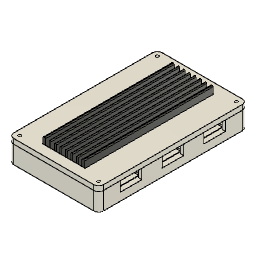
TLSmootherBox_v17 (Autodesk Fusion 360 design; units mm, degrees)
Autodesk Fusion 360 part; units mm, degrees
sketch "Sketch1" plane through (0, 0, 0) normal (0, 0, 1) x (1, 0, 0) in component "Base"
  line L0 (0, 108.9935) -> (0, -108.9935) construction
  line L1 (-168.2514, 0) -> (168.2514, 0) construction
  line L2 (37.875, 24.125) -> (-37.875, 24.125)
  line L3 (-37.875, 24.125) -> (-37.875, -24.125)
  line L4 (-37.875, -24.125) -> (37.875, -24.125)
  line L5 (37.875, -24.125) -> (37.875, 24.125)
  line L6 (37.875, 24.125) -> (-37.875, -24.125) construction
  line L7 (-37.875, 24.125) -> (37.875, -24.125) construction
  line L8 (-42.875, 25.125) -> (42.875, 25.125)
  line L9 (42.875, 25.125) -> (42.875, -25.125)
  line L10 (42.875, -25.125) -> (-42.875, -25.125)
  line L11 (-42.875, -25.125) -> (-42.875, 25.125)
  line L12 (44.875, -27.125) -> (-44.875, -27.125)
  line L13 (-44.875, -27.125) -> (-44.875, 27.125)
  line L14 (-44.875, 27.125) -> (44.875, 27.125)
  line L15 (44.875, 27.125) -> (44.875, -27.125)
  circle A0 centre (-41.625, 23.875) radius 0.875
  circle A1 centre (41.625, 23.875) radius 0.875
  circle A2 centre (-41.625, -23.875) radius 0.875
  circle A3 centre (41.625, -23.875) radius 0.875
  line L16 (-44.875, 27.125) -> (-38.875, 27.125)
  line L17 (-38.875, 27.125) -> (-38.875, 21.125)
  line L18 (-38.875, 21.125) -> (-44.875, 21.125)
  line L19 (-44.875, 21.125) -> (-44.875, 27.125)
  line L20 (38.875, 21.125) -> (44.875, 21.125)
  line L21 (38.875, 27.125) -> (38.875, 21.125)
  line L22 (-38.875, -21.125) -> (-44.875, -21.125)
  line L23 (-38.875, -27.125) -> (-38.875, -21.125)
  line L24 (38.875, -27.125) -> (38.875, -21.125)
  line L25 (38.875, -21.125) -> (44.875, -21.125)
  line L26 (-37.875, 22.125) -> (37.875, 22.125)
  line L27 (-37.875, -22.125) -> (37.875, -22.125)
  line L28 (-35.875, 24.125) -> (-35.875, -24.125)
  line L29 (-12.625, 24.125) -> (-12.625, -24.125)
  line L30 (-14.625, 24.125) -> (-14.625, -24.125)
  circle A4 centre (-41.625, 23.875) radius 1.25
  circle A5 centre (41.625, 23.875) radius 1.25
  circle A6 centre (-41.625, -23.875) radius 1.25
  circle A7 centre (41.625, -23.875) radius 1.25
  dimension "d9" = 48.25
  dimension "d11" = 75.75
  dimension "d14" = 1
  dimension "d15" = 5
  dimension "d36" = 1.75
  dimension "d83" = 0
  dimension "d84" = 0
  dimension "d85" = 0
  dimension "d86" = 0
  dimension "d95" = 0
  dimension "d96" = 0
  dimension "d97" = 0
  dimension "d98" = 0
  dimension "d103" = 0
  dimension "d104" = 0
  dimension "d105" = 0
  dimension "d106" = 0
  dimension "d134" = 0
  dimension "d135" = 0
  dimension "d136" = 0
  dimension "d137" = 0
  dimension "d147" = 21.125
  dimension "d148" = 38.875
  dimension "d149" = 41.625
  dimension "d150" = 23.875
  dimension "d154" = 2
  dimension "d160" = 2
  dimension "d161" = 25.25
  dimension "d162" = 2
  dimension "d188" = 0
  dimension "d189" = 0
  dimension "d190" = 0
  dimension "d191" = 0
  dimension "d240" = 2.5
  constraint horizontal L1
  constraint perpendicular L2 L3
  constraint parallel L2 L4
  constraint parallel L3 L5
  constraint horizontal L2
  constraint coincident L6 origin
  constraint coincident L7 origin
  constraint horizontal L8
  constraint vertical L9
  constraint horizontal L10
  constraint vertical L11
  constraint symmetric L1 L8 L10
  constraint symmetric L0 L9 L11
  constraint midpoint L0 origin
  constraint midpoint origin L1
  constraint symmetric L0 A0 A1
  constraint symmetric L1 A0 A2
  constraint symmetric L1 A1 A3
  constraint horizontal L16
  constraint vertical L17
  constraint horizontal L18
  constraint vertical L19
  constraint symmetric L0 L16.end L21.start
  constraint symmetric L0 L17.end L20.start
  constraint symmetric L0 L18.end L20.end
  constraint symmetric L1 L16.end L23.start
  constraint symmetric L1 L17.end L22.start
  constraint symmetric L1 L18.end L22.end
  constraint symmetric L1 L20.start L24.end
  constraint symmetric L1 L20.end L25.end
  constraint symmetric L1 L21.start L24.start
  constraint coincident L3 L26.start
  constraint coincident L5 L26.end
  constraint perpendicular L5 L26
  constraint coincident L3 L27.start
  constraint coincident L5 L27.end
  constraint perpendicular L5 L27
  constraint symmetric L1 L26 L27
  constraint coincident L2 L28.start
  constraint coincident L4 L28.end
  constraint perpendicular L4 L28
  constraint coincident L2 L29.start
  constraint coincident L4 L29.end
  constraint perpendicular L4 L29
  constraint coincident L2 L30.start
  constraint coincident L4 L30.end
  constraint perpendicular L4 L30
  constraint concentric A0 A4
  constraint symmetric L0 A4 A5
  constraint symmetric L1 A4 A6
  constraint symmetric L1 A5 A7
  measures "d9" distance of L2 L4
  measures "d11" distance of L3 L5
  measures "d14" distance of L2 L8
  measures "d15" distance of L3 L11
  measures "d36" diameter of A0
  measures "d147" distance of L1 L18
  measures "d148" distance of L0 L17
  measures "d149" distance of L0 A0.centre
  measures "d150" distance of L1 A0.centre
  measures "d154" distance of L2 L26
  measures "d160" distance of L3 L28
  measures "d161" distance of L3 L29
  measures "d162" distance of L29 L30
  measures "d240" diameter of A4
extrude "Extrude1" add sketch "Sketch1" along normal blind 2 contours L2 L5 L26 L29 | L2 L26 L29 L30 | L5 L26 L27 L29 | L2 L26 L28 L30 | L26 L27 L29 L30 | L4 L5 L27 L29 | L2 L3 L26 L28 | L26 L27 L28 L30 | L4 L27 L29 L30 | L3 L26 L27 L28 | L4 L27 L28 L30 | L3 L4 L27 L28 | L8 L11 L13 L14 L16 L17 L18 L19 | L8 L11 A4 | L8 L11 L17 L18 A4 | A4 | L8 L14 L17 L21 | L8 L9 L10 L11 L17 L18 L20 L21 L22 L23 L24 L25 | L11 L13 L18 L22 | L8 L9 L14 L15 L20 L21 | L8 L9 L20 L21 A5 | L10 L11 L22 L23 A6 | L10 L11 L12 L13 L22 L23 | L8 L9 A5 | A5 | L10 L11 A6 | A6 | L9 L15 L20 L25 | L10 L12 L23 L24 | L9 L10 L12 L15 L24 L25 | L9 L10 L24 L25 A7 | A7 | L9 L10 A7 | A0 | A1 | A2 | A3 makes body 1 in component "Base"
extrude "Extrude2" add sketch "Sketch1" along normal blind 10.75 contours L8 L11 L13 L14 L16 L17 L18 L19 | L8 L11 A4 | L8 L11 L17 L18 A4 | A4 | L8 L14 L17 L21 | L11 L13 L18 L22 | L8 L9 L14 L15 L20 L21 | L8 L9 L20 L21 A5 | L10 L11 L22 L23 A6 | L10 L11 L12 L13 L22 L23 | L8 L9 A5 | A5 | L10 L11 A6 | A6 | L9 L15 L20 L25 | L10 L12 L23 L24 | L9 L10 L12 L15 L24 L25 | L9 L10 L24 L25 A7 | A7 | L9 L10 A7 | A0 | A1 | A2 | A3 bodies 1 in component "Base"
extrude "Extrude5" cut sketch "Sketch1" against normal blind 6 from surface at 10.75 contours A4 | A5 | A6 | A7 | A0 | A1 | A2 | A3 bodies 1 in component "Base"
extrude "Extrude4" add sketch "Sketch1" along normal blind 2.75 from surface at 2 contours L8 L11 A4 | L8 L11 L17 L18 A4 | A4 | L8 L9 L10 L11 L17 L18 L20 L21 L22 L23 L24 L25 | L8 L9 L20 L21 A5 | L10 L11 L22 L23 A6 | L8 L9 A5 | A5 | L10 L11 A6 | A6 | L9 L10 L24 L25 A7 | A7 | L9 L10 A7 | A0 | A1 | A2 | A3 bodies 1 in component "Base"
extrude "Extrude3" add sketch "Sketch1" along normal blind 1 from surface at 2 contours L2 L26 L29 L30 | L2 L26 L28 L30 | L26 L27 L29 L30 | L2 L3 L26 L28 | L4 L27 L29 L30 | L3 L26 L27 L28 | L4 L27 L28 L30 | L3 L4 L27 L28 bodies 1 in component "Base"
pattern_linear "R-Pattern2" count 3 spacing 25.25 along (1, 0, 0) of "Extrude3" in component "Base"
fillet "Fillet1" radius 3 4 edges at (44.875, -27.125, 5.375) (-44.875, -27.125, 5.375) (-44.875, 27.125, 5.375) (44.875, 27.125, 5.375) on bodies 1 in component "Base"
fillet "Fillet2" radius 2 4 edges at (-38.875, 21.125, 7.75) (38.875, 21.125, 7.75) (-38.875, -21.125, 7.75) (38.875, -21.125, 7.75) on bodies 1 in component "Base"
fillet "Fillet3" radius 0.5 8 edges at (-42.875, -21.125, 7.75) (-38.875, -25.125, 7.75) (38.875, -25.125, 7.75) (42.875, -21.125, 7.75) (38.875, 25.125, 7.75) (42.875, 21.125, 7.75) (-42.875, 21.125, 7.75) (-38.875, 25.125, 7.75) on bodies 1 in component "Base"
sketch "Sketch2" plane through (0, -27.125, 0) normal (0, -1, 0) x (1, 0, 0) in component "Base"
  line L0 (-41.875, 10.75) -> (-41.875, 0)
  line L1 (-41.875, 0) -> (41.875, 0)
  line L2 (41.875, 0) -> (41.875, 10.75)
  line L3 (41.875, 10.75) -> (-41.875, 10.75)
  line L4 (0, 68.7375) -> (0, -68.7375) construction
  line L5 (37.875, 3) -> (-37.875, 3)
  line L6 (-37.875, 3) -> (-37.875, 4.75)
  line L7 (-37.875, 4.75) -> (37.875, 4.75)
  line L8 (37.875, 4.75) -> (37.875, 3)
  line L9 (-31.75, 10.75) -> (-31.75, 4.75)
  line L10 (-18.75, 10.75) -> (-18.75, 4.75)
  dimension "d167" = 6.125
  dimension "d168" = 13
  constraint vertical L4
  constraint midpoint L4 origin
  constraint coincident L3 L9.start
  constraint coincident L7 L9.end
  constraint perpendicular L7 L9
  constraint coincident L3 L10.start
  constraint coincident L7 L10.end
  constraint perpendicular L7 L10
  measures "d167" distance of L6 L9
  measures "d168" distance of L9 L10
extrude "Extrude6" cut sketch "Sketch2" against normal through all contours L3 L7 L9 L10 bodies 1 in component "Base"
pattern_linear "R-Pattern1" count 3 spacing 25.25 along (1, 0, 0) of "Extrude6" in component "Base"
sketch "Sketch1 (2)" plane through (0, 0, 2) normal (0, 0, 1) x (1, 0, 0) in component "Lid"
  line L0 (-31.75, 27.125) -> (-41.875, 27.125)
  arc A0 (-41.875, 27.125) -> (-44.875, 24.125) centre (-41.875, 24.125) ccw
  line L1 (-44.875, 24.125) -> (-44.875, -24.125)
  arc A1 (-44.875, -24.125) -> (-41.875, -27.125) centre (-41.875, -24.125) ccw
  line L2 (-41.875, -27.125) -> (-31.75, -27.125)
  line L3 (-31.75, -25.125) -> (-38.375, -25.125)
  line L4 (-42.875, -20.625) -> (-42.875, 20.625)
  line L5 (-38.375, 25.125) -> (-31.75, 25.125)
  line L6 (31.75, -27.125) -> (41.875, -27.125)
  arc A2 (41.875, -27.125) -> (44.875, -24.125) centre (41.875, -24.125) ccw
  line L7 (44.875, -24.125) -> (44.875, 24.125)
  arc A3 (44.875, 24.125) -> (41.875, 27.125) centre (41.875, 24.125) ccw
  line L8 (41.875, 27.125) -> (31.75, 27.125)
  line L9 (31.75, 25.125) -> (38.375, 25.125)
  line L10 (42.875, 20.625) -> (42.875, -20.625)
  line L11 (38.375, -25.125) -> (31.75, -25.125)
  line L12 (31.75, -25.125) -> (38.375, -25.125)
  line L13 (42.875, -20.625) -> (42.875, 20.625)
  line L14 (-42.875, 20.625) -> (-42.875, -20.625)
  line L15 (0, 108.9935) -> (0, -108.9935) construction
  line L16 (-168.2514, 0) -> (168.2514, 0) construction
  line L17 (37.875, -24.125) -> (37.875, 24.125)
  line L18 (37.875, 24.125) -> (-37.875, 24.125)
  line L19 (-37.875, 24.125) -> (-37.875, -24.125)
  line L20 (-37.875, -24.125) -> (37.875, -24.125)
  arc A4 (-38.875, -24.625) -> (-38.375, -25.125) centre (-38.375, -24.625) ccw
  line L21 (-38.875, -24.625) -> (-38.875, -23.125)
  arc A5 (-38.875, -23.125) -> (-40.875, -21.125) centre (-40.875, -23.125) ccw
  line L22 (-40.875, -21.125) -> (-42.375, -21.125)
  arc A6 (-42.875, -20.625) -> (-42.375, -21.125) centre (-42.375, -20.625) ccw
  arc A7 (-42.375, 21.125) -> (-42.875, 20.625) centre (-42.375, 20.625) ccw
  line L23 (-42.375, 21.125) -> (-40.875, 21.125)
  arc A8 (-40.875, 21.125) -> (-38.875, 23.125) centre (-40.875, 23.125) ccw
  line L24 (-38.875, 23.125) -> (-38.875, 24.625)
  arc A9 (-38.375, 25.125) -> (-38.875, 24.625) centre (-38.375, 24.625) ccw
  arc A10 (38.875, 24.625) -> (38.375, 25.125) centre (38.375, 24.625) ccw
  line L25 (38.875, 24.625) -> (38.875, 23.125)
  arc A11 (38.875, 23.125) -> (40.875, 21.125) centre (40.875, 23.125) ccw
  line L26 (40.875, 21.125) -> (42.375, 21.125)
  arc A12 (42.875, 20.625) -> (42.375, 21.125) centre (42.375, 20.625) ccw
  arc A13 (42.375, -21.125) -> (42.875, -20.625) centre (42.375, -20.625) ccw
  line L27 (42.375, -21.125) -> (40.875, -21.125)
  arc A14 (40.875, -21.125) -> (38.875, -23.125) centre (40.875, -23.125) ccw
  line L28 (38.875, -23.125) -> (38.875, -24.625)
  arc A15 (38.375, -25.125) -> (38.875, -24.625) centre (38.375, -24.625) ccw
  arc A16 (-38.375, 25.125) -> (-38.875, 24.625) centre (-38.375, 24.625) ccw
  line L29 (-38.875, 24.625) -> (-38.875, 23.125)
  arc A17 (-40.875, 21.125) -> (-38.875, 23.125) centre (-40.875, 23.125) ccw
  line L30 (-40.875, 21.125) -> (-42.375, 21.125)
  arc A18 (-42.375, 21.125) -> (-42.875, 20.625) centre (-42.375, 20.625) ccw
  arc A19 (-42.875, -20.625) -> (-42.375, -21.125) centre (-42.375, -20.625) ccw
  line L31 (-42.375, -21.125) -> (-40.875, -21.125)
  arc A20 (-38.875, -23.125) -> (-40.875, -21.125) centre (-40.875, -23.125) ccw
  line L32 (-38.875, -23.125) -> (-38.875, -24.625)
  arc A21 (-38.875, -24.625) -> (-38.375, -25.125) centre (-38.375, -24.625) ccw
  arc A22 (38.375, -25.125) -> (38.875, -24.625) centre (38.375, -24.625) ccw
  line L33 (38.875, -24.625) -> (38.875, -23.125)
  arc A23 (40.875, -21.125) -> (38.875, -23.125) centre (40.875, -23.125) ccw
  line L34 (40.875, -21.125) -> (42.375, -21.125)
  arc A24 (42.375, -21.125) -> (42.875, -20.625) centre (42.375, -20.625) ccw
  arc A25 (42.875, 20.625) -> (42.375, 21.125) centre (42.375, 20.625) ccw
  line L35 (42.375, 21.125) -> (40.875, 21.125)
  arc A26 (38.875, 23.125) -> (40.875, 21.125) centre (40.875, 23.125) ccw
  line L36 (38.875, 23.125) -> (38.875, 24.625)
  arc A27 (38.875, 24.625) -> (38.375, 25.125) centre (38.375, 24.625) ccw
  line L37 (-38.875, 27.125) -> (-38.875, -27.125)
  line L38 (38.875, 27.125) -> (38.875, -27.125)
  line L39 (-44.875, 13) -> (44.875, 13)
  line L40 (-44.875, -13) -> (44.875, -13)
  line L41 (-42.375, 13) -> (-42.375, -13)
  line L42 (42.375, 13) -> (42.375, -13)
  line L43 (-31.75, 25.125) -> (-31.75, 27.125)
  line L44 (-31.75, -27.125) -> (-31.75, -25.125)
  line L45 (31.75, -25.125) -> (31.75, -27.125)
  line L46 (31.75, 27.125) -> (31.75, 25.125)
  line L47 (31.75, 25.125) -> (31.75, 27.125)
  line L48 (18.75, 27.125) -> (18.75, 25.125)
  line L49 (18.75, 25.125) -> (6.5, 25.125)
  line L50 (6.5, 25.125) -> (6.5, 27.125)
  line L51 (6.5, 27.125) -> (-6.5, 27.125)
  line L52 (-6.5, 27.125) -> (-6.5, 25.125)
  line L53 (-6.5, 25.125) -> (-18.75, 25.125)
  line L54 (-18.75, 25.125) -> (-18.75, 27.125)
  line L55 (-18.75, 27.125) -> (-31.75, 27.125)
  line L56 (-31.75, 27.125) -> (-31.75, 25.125)
  line L57 (-31.75, 25.125) -> (-38.375, 25.125)
  line L58 (-38.375, -25.125) -> (-31.75, -25.125)
  line L59 (-31.75, -25.125) -> (-31.75, -27.125)
  line L60 (-18.75, -27.125) -> (-18.75, -25.125)
  line L61 (-18.75, -25.125) -> (-6.5, -25.125)
  line L62 (-6.5, -25.125) -> (-6.5, -27.125)
  line L63 (-6.5, -27.125) -> (6.5, -27.125)
  line L64 (6.5, -27.125) -> (6.5, -25.125)
  line L65 (6.5, -25.125) -> (18.75, -25.125)
  line L66 (18.75, -25.125) -> (18.75, -27.125)
  line L67 (18.75, -27.125) -> (31.75, -27.125)
  line L68 (31.75, -27.125) -> (31.75, -25.125)
  line L69 (35.875, 22.125) -> (35.875, -22.125)
  line L70 (35.875, -22.125) -> (14.625, -22.125)
  line L71 (14.625, -22.125) -> (14.625, 22.125)
  line L72 (14.625, 22.125) -> (35.875, 22.125)
  line L73 (10.625, 22.125) -> (10.625, -22.125)
  line L74 (10.625, -22.125) -> (-10.625, -22.125)
  line L75 (-10.625, -22.125) -> (-10.625, 22.125)
  line L76 (-10.625, 22.125) -> (10.625, 22.125)
  line L77 (-14.625, 22.125) -> (-14.625, -22.125)
  line L78 (-14.625, -22.125) -> (-35.875, -22.125)
  line L79 (-35.875, -22.125) -> (-35.875, 22.125)
  line L80 (-35.875, 22.125) -> (-14.625, 22.125)
  line L81 (-6.5, 27.125) -> (-18.75, 27.125)
  line L82 (18.75, 27.125) -> (6.5, 27.125)
  line L83 (-31.75, 27.125) -> (-18.75, 27.125)
  line L84 (-6.5, 27.125) -> (6.5, 27.125)
  line L85 (18.75, 27.125) -> (31.75, 27.125)
  line L86 (-18.75, -27.125) -> (-31.75, -27.125)
  line L87 (-18.75, -27.125) -> (-6.5, -27.125)
  line L88 (6.5, -27.125) -> (-6.5, -27.125)
  line L89 (6.5, -27.125) -> (18.75, -27.125)
  line L90 (31.75, -27.125) -> (18.75, -27.125)
  line L91 (-31.75, 25.125) -> (31.75, 25.125)
  line L92 (-31.75, -25.125) -> (31.75, -25.125)
  circle A28 centre (41.625, 23.875) radius 0.875
  circle A29 centre (-41.625, 23.875) radius 0.875
  circle A30 centre (-41.625, -23.875) radius 0.875
  circle A31 centre (41.625, -23.875) radius 0.875
  dimension "d87" = 0
  dimension "d88" = 0
  dimension "d89" = 0
  dimension "d90" = 0
  dimension "d99" = 0
  dimension "d100" = 0
  dimension "d101" = 0
  dimension "d102" = 0
  dimension "d107" = 0
  dimension "d108" = 0
  dimension "d109" = 0
  dimension "d110" = 0
  dimension "d113" = 1
  dimension "d123" = 26
  dimension "d124" = 0.5
  dimension "d138" = 0
  dimension "d139" = 0
  dimension "d140" = 0
  dimension "d141" = 0
  dimension "d192" = 0
  dimension "d193" = 0
  dimension "d194" = 0
  dimension "d195" = 0
  dimension "d215" = 84.75
  dimension "d216" = 85.75
  dimension "d217" = 77.75
  dimension "d218" = 3.5
  constraint coincident L0 L37.start
  constraint coincident L2 L37.end
  constraint perpendicular L2 L37
  constraint coincident L8 L38.start
  constraint coincident L6 L38.end
  constraint perpendicular L6 L38
  constraint coincident L1 L39.start
  constraint coincident L7 L39.end
  constraint perpendicular L7 L39
  constraint coincident L1 L40.start
  constraint coincident L7 L40.end
  constraint perpendicular L7 L40
  constraint symmetric L16 L39 L40
  constraint coincident L39 L41.start
  constraint coincident L40 L41.end
  constraint perpendicular L40 L41
  constraint coincident L39 L42.start
  constraint coincident L40 L42.end
  constraint perpendicular L40 L42
  constraint symmetric L15 L41 L42
  constraint coincident L5.end L43.start
  constraint coincident L9.start L46.end
  constraint coincident L3.start L44.end
  constraint coincident L11.end L12.start
  measures "d113" distance of L19 L37
  measures "d123" distance of L39 L40
  measures "d124" distance of L4 L41
  measures "d215" distance of L41 L42
  measures "d216" distance of L4 L13
  measures "d217" distance of L37 L38
  measures "d218" distance of L37 L41
extrude "Extrude1'" add sketch "Sketch1 (2)" along normal blind 2 separate body contours L0 L5 A9 A16 L37 L43 L56 L57 | L43 L54 L55 L56 L83 L91 | L0 A0 L1 L4 L14 A7 L23 A8 L24 L29 A17 L30 A18 L37 L39 | L5 L9 L17 L18 L19 L24 A9 A10 L25 A16 L29 L36 A27 L37 L38 L39 L49 L53 L57 L91 | L52 L53 L54 L81 L91 | L50 L51 L52 L84 L91 | L4 L14 A7 L23 A8 A17 L30 A18 L37 L39 | L48 L49 L50 L82 L91 | L1 L4 L14 L39 L40 | L37 L39 L40 L41 | L46 L47 L48 L85 L91 | L1 A1 L2 L4 L14 L21 A5 L22 A6 A19 L31 A20 L32 L37 L40 | L4 L14 L39 L40 L41 | L3 L11 L12 L17 L19 L20 A4 L21 L28 A15 L32 A21 A22 L33 L37 L38 L40 L58 L61 L65 L92 | L4 L14 A5 L22 A6 A19 L31 A20 L37 L40 | L17 L18 L19 L39 L69 L71 L72 L73 L75 L76 L77 L79 L80 | L8 L9 A10 A27 L38 L46 L47 | L17 L19 L20 L40 L69 L70 L71 L73 L74 L75 L77 L78 L79 | L39 L77 L79 L80 | L7 A3 L8 L10 L13 L25 A11 L26 A12 A25 L35 A26 L36 L38 L39 | L2 L3 A4 A21 L37 L44 L58 L59 | L40 L77 L78 L79 | L39 L73 L75 L76 | L10 L13 A11 L26 A12 A25 L35 A26 L38 L39 | L44 L59 L60 L86 L92 | L40 L73 L74 L75 | L39 L69 L71 L72 | L38 L39 L40 L42 | L7 L10 L13 L39 L40 | L60 L61 L62 L87 L92 | L40 L69 L70 L71 | L10 L13 A13 L27 A14 A23 L34 A24 L38 L40 | L10 L13 L39 L40 L42 | L6 A2 L7 L10 L13 A13 L27 A14 L28 L33 A23 L34 A24 L38 L40 | L62 L63 L64 L88 L92 | L64 L65 L66 L89 L92 | L6 L11 L12 A15 A22 L38 L45 L68 | L45 L66 L67 L68 L90 L92 | A28 | A29 | A30 | A31 makes body 2 in component "Lid"
extrude "Extrude2'" add sketch "Sketch1 (2)" along normal blind 1 from surface at 2 contours L0 L5 A9 A16 L37 L43 L56 L57 | L43 L54 L55 L56 L83 L91 | L0 A0 L1 L4 L14 A7 L23 A8 L24 L29 A17 L30 A18 L37 L39 | L52 L53 L54 L81 L91 | L50 L51 L52 L84 L91 | L48 L49 L50 L82 L91 | L1 L4 L14 L39 L40 | L46 L47 L48 L85 L91 | L1 A1 L2 L4 L14 L21 A5 L22 A6 A19 L31 A20 L32 L37 L40 | L8 L9 A10 A27 L38 L46 L47 | L7 A3 L8 L10 L13 L25 A11 L26 A12 A25 L35 A26 L36 L38 L39 | L2 L3 A4 A21 L37 L44 L58 L59 | L44 L59 L60 L86 L92 | L7 L10 L13 L39 L40 | L60 L61 L62 L87 L92 | L6 A2 L7 L10 L13 A13 L27 A14 L28 L33 A23 L34 A24 L38 L40 | L62 L63 L64 L88 L92 | L64 L65 L66 L89 L92 | L6 L11 L12 A15 A22 L38 L45 L68 | L45 L66 L67 L68 L90 L92 | A28 | A29 | A30 | A31 bodies 2 in component "Lid"
extrude "Extrude6'" cut sketch "Sketch1 (2)" along normal through all contours A28 | A29 | A30 | A31 bodies 2 in component "Lid"
extrude "Extrude4'" add sketch "Sketch1 (2)" along normal blind 1 from surface at 2 contours L4 L14 A7 L23 A8 A17 L30 A18 L37 L39 | L37 L39 L40 L41 | L4 L14 L39 L40 L41 | L4 L14 A5 L22 A6 A19 L31 A20 L37 L40 | L10 L13 A11 L26 A12 A25 L35 A26 L38 L39 | L38 L39 L40 L42 | L10 L13 A13 L27 A14 A23 L34 A24 L38 L40 | L10 L13 L39 L40 L42 bodies 2 in component "Lid"
extrude "Extrude5'" add sketch "Sketch1 (2)" along normal blind 1.5 from surface at 3 contours L37 L39 L40 L41 | L38 L39 L40 L42 bodies 2 in component "Lid"
fillet "Fillet4" radius 0.5 8 edges at (-42.375, -13, 5.75) (-38.875, -13, 5.75) (-42.375, 13, 5.75) (-38.875, 13, 5.75) (38.875, 13, 5.75) (42.375, 13, 5.75) (38.875, -13, 5.75) (42.375, -13, 5.75) on bodies 2 in component "Lid"
sketch "Sketch3" plane through (0, 0, 2) normal (0, 0, 1) x (1, 0, 0) in component "Lid"
  line L0 (-31.75, 27.125) -> (-18.75, 27.125)
  line L1 (-31.75, 25.125) -> (-31.75, 27.125)
  line L2 (-18.75, 25.125) -> (-18.75, 27.125)
  line L3 (37.875, 24.125) -> (-37.875, 24.125)
  line L4 (-37.875, 24.125) -> (-37.875, -24.125)
  line L5 (-37.875, -24.125) -> (37.875, -24.125)
  line L6 (37.875, -24.125) -> (37.875, 24.125)
  line L7 (-31.75, 27.125) -> (-31.75, 16.125)
  line L8 (-31.75, 16.125) -> (-18.75, 16.125)
  line L9 (-18.75, 16.125) -> (-18.75, 27.125)
  line L10 (0, 108.9935) -> (0, -108.9935) construction
  line L11 (-168.2514, 0) -> (168.2514, 0) construction
  dimension "d172" = 8
  constraint coincident L0 L1.end
  constraint perpendicular L3 L7
  constraint perpendicular L7 L8
  constraint coincident L0 L2.end
  constraint perpendicular L0 L9
  constraint coincident L1.start L7
  constraint coincident L2.start L9
  measures "d172" distance of L3 L8
extrude "Extrude7" add sketch "Sketch3" along normal blind 1 from surface at 2 contours L0 L1 L2 L3 L7 L9 | L3 L7 L8 L9 bodies 2 in component "Lid"
fillet "Fillet3'" radius 0.5 2 edges at (-31.75, 16.125, 4.5) (-18.75, 16.125, 4.5) on bodies 2 in component "Lid"
mirror "Mirror2" about plane through (0, 0, 0) normal (0, 1, 0) of "Extrude7", "Fillet3'" in component "Lid"
pattern_linear "R-Pattern2'" count 3 spacing 25.25 along (1, 0, 0) of "Extrude7", "Fillet3'", "Mirror2" in component "Lid"
sketch "Sketch1 (3)" plane through (0, 0, 0) normal (0, 0, 1) x (1, 0, 0) in component "HeatSink"
  line L0 (0, 40.2668) -> (0, -40.2668) construction
  line L1 (-54, 0) -> (54, 0) construction
  line L2 (-12.5, 0) -> (12.5, 0)
  line L3 (12.5, 0) -> (12.5, 10)
  line L4 (12.5, 10) -> (-12.5, 10)
  line L5 (-12.5, 10) -> (-12.5, 0)
  line L6 (-1.075, 10) -> (1.075, 10)
  line L7 (1.075, 10) -> (1.075, 1.5)
  line L8 (1.075, 1.5) -> (-1.075, 1.5)
  line L9 (-1.075, 1.5) -> (-1.075, 10)
  dimension "d199" = 25
  dimension "d200" = 10
  dimension "d201" = 2.15
  dimension "d202" = 1.5
  constraint horizontal L1
  constraint midpoint origin L1
  constraint vertical L0
  constraint midpoint origin L0
  constraint horizontal L2
  constraint vertical L3
  constraint horizontal L4
  constraint vertical L5
  constraint coincident L1 L2.start
  constraint symmetric L0 L3 L5
  constraint horizontal L6
  constraint vertical L7
  constraint horizontal L8
  constraint vertical L9
  constraint coincident L4 L6.start
  measures "d199" distance of L3 L5
  measures "d200" distance of L2 L4
  measures "d201" distance of L7 L9
  measures "d202" distance of L2 L8
extrude "Extrude1''" add sketch "Sketch1 (3)" along normal blind 84.75 separate body makes body 3 in component "HeatSink"
extrude "Extrude2''" cut sketch "Sketch1 (3)" along normal through all contours L4 L6 L7 L8 L9 bodies 3 in component "HeatSink"
fillet "Fillet1'" radius 1 2 edges at (-1.075, 1.5, 42.375) (1.075, 1.5, 42.375) on bodies 3 in component "HeatSink"
fillet "Fillet2'" radius 0.5 2 edges at (1.075, 10, 42.375) (-1.075, 10, 42.375) on bodies 3 in component "HeatSink"
pattern_linear "R-Pattern1'" count 7 spacing 3.3 along (-1, 0, 0) both ways of "Extrude2''", "Fillet1'", "Fillet2'" in component "HeatSink"
fillet "Fillet4'" radius 0.2 2 edges at (-12.5, 0, 42.375) (12.5, 0, 42.375) on bodies 3 in component "HeatSink"
fillet "Fillet5" radius 0.5 2 edges at (-12.5, 10, 42.375) (12.5, 10, 42.375) on bodies 3 in component "HeatSink"
sketch "Sketch2 (2)" plane through (-12.5, 0, 0) normal (-1, 0, 0) x (0, 0, 1) in component "HeatSink"
  line L0 (84.75, 9.5) -> (0, 9.5)
  line L1 (0, 9.5) -> (0, 0.2)
  line L2 (0, 0.2) -> (84.75, 0.2)
  line L3 (84.75, 0.2) -> (84.75, 9.5)
  line L4 (0, 40.2668) -> (0, -40.2668)
  line L5 (0, 1.49) -> (3.5, 1.49)
  line L6 (3.5, 1.49) -> (3.5, 10)
  line L7 (3.5, 10) -> (0, 10)
  line L8 (0, 10) -> (0, 1.49)
  line L9 (-93.0925, 0) -> (93.0925, 0) construction
  line L10 (84.75, 28.7) -> (84.75, -28.3) construction
  line L11 (84.75, 1.49) -> (81.25, 1.49)
  line L12 (81.25, 1.49) -> (81.25, 10)
  line L13 (81.25, 10) -> (84.75, 10)
  line L14 (84.75, 10) -> (84.75, 1.49)
  dimension "d220" = 3.5
  dimension "d221" = 1.49
  dimension "d222" = 10
  dimension "d224" = 3.5
  dimension "d225" = 10
  dimension "d226" = 1.49
  constraint horizontal L5
  constraint vertical L6
  constraint horizontal L7
  constraint vertical L8
  constraint coincident L4 L5.start
  constraint parallel L2 L9
  constraint midpoint L9 origin
  constraint vertical L10
  constraint midpoint L2.end L10
  constraint horizontal L11
  constraint vertical L12
  constraint horizontal L13
  constraint vertical L14
  constraint coincident L10 L11.start
  measures "d220" distance of L4 L6
  measures "d221" distance of L5 L9
  measures "d222" distance of L7 L9
  measures "d224" distance of L10 L12
  measures "d225" distance of L9 L13
  measures "d226" distance of L9 L11
extrude "Extrude3'" cut sketch "Sketch2 (2)" against normal through all contours L0 L1 L4 L5 L6 L8 | L0 L4 L6 L7 L8 bodies 3 in component "HeatSink"
extrude "Extrude4''" cut sketch "Sketch2 (2)" against normal through all contours L0 L3 L11 L12 L14 | L0 L12 L13 L14 bodies 3 in component "HeatSink"
chamfer "Chamfer1" [suppressed] in component "Lid"
component "Base" placed x (0, 0, -1) y (-1, 0, 0) z (0, 1, 0) at (0, -7.76, 42.375)
component "Lid" placed x (0, 0, -1) y (1, 0, 0) z (0, -1, 0) at (0, 7.99, 42.375)
component "HeatSink" placed x (1, 0, 0) y (0, 1, 0) z (0, 0, 1) at (0, 0, 0)
equation "Slots = 3"
equation "Wpcb = 25.25 mm"
equation "Lpcb = 48.25 mm"
equation "Hpcb = 7.75 mm"
equation "Wall = 2 mm"
equation "d9 = Lpcb"
equation "d11 = Wpcb * Slots"
equation "d14 = Hspace"
equation "d15 = Vspace"
equation "d16 = -Wall"
equation "d17 = Wall"
equation "BaseHeight = Wall + Tbasement + Hpcb"
equation "LidHeight = 1 mm"
equation "d21 = BaseHeight"
equation "d25 = Tbasement"
equation "Tpcb = 1.75 mm"
equation "Tbasement = 1 mm"
equation "d29 = Tbasement + Tpcb"
equation "d45 = Slots"
equation "d47 = Wpcb"
equation "d64 = Wall"
equation "d66 = LidHeight"
equation "d115 = LidHeight"
equation "Tsupport = 1.5 mm"
equation "d121 = Tsupport"
equation "Vspace = 5 mm"
equation "Hspace = 1 mm"
equation "Wbase = Slots * Wpcb + 2 * Vspace + 2 * Wall"
equation "Hbase = Lpcb + 2 * Hspace + 2 * Wall"
equation "d147 = Hbase / 2 - Corner"
equation "d148 = Wbase / 2 - Corner"
equation "d149 = Wbase / 2 - HoleDist"
equation "d150 = Hbase / 2 - HoleDist"
equation "HoleDist = 3.25 mm"
equation "Corner = 6 mm"
equation "d161 = Wpcb"
equation "d163 = Slots"
equation "d165 = Wpcb"
equation "d167 = ( Wpcb - 13 mm ) / 2"
equation "d174 = LidHeight"
equation "d184 = -Wpcb"
